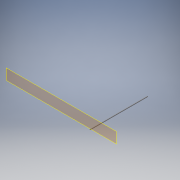
# Autodesk Inventor part: Part9
Saved by Autodesk Inventor 2016 (Build 200138000, 138)
## iProperties
Created: 2016-01-25
Part Number: Part9
Material: Generic
Document SubType Name: Modeling
Designer: ares-b02
Density: 1 g/cm^3
Appearance: Default
Author: ares-b02
Autodesk Inventor part; units mm, degrees
ref_plane "YZ Plane" through (0, 0, 0) normal (1, 0, 0) x (0, 1, 0)
ref_plane "XZ Plane" through (0, 0, 0) normal (0, 1, 0) x (-1, 0, 0)
ref_plane "XY Plane" through (0, 0, 0) normal (0, 0, 1) x (1, 0, 0)
ref_plane "Work Plane1" through (1008.1734, -842.2122, 0) normal (0, 0, 1) x (0.8815, 0.4723, 0)
sketch "Sketch1" plane through (1008.1734, -842.2122, 0) normal (0, 0, 1) x (0.8815, 0.4723, 0)
  circle A0 centre (-201.7533, -7.3155) radius 3.175
  point P0 (-490.9201, 1218.496)
  dimension "d0" = 6.35
  constraints: 1 centre point
  measures "d0" diameter of A0
extrude "Extrusion1" add sketch "Sketch1" against normal blind 703.1228
body "Solid1"
